Autodesk Inventor part; units mm, degrees
(part 2 of 2)
sketch "Sketch8" plane through (0, 0, 0) normal (0, 0, -1) x (-1, 0, 0)
  circle A0 centre (-9.53986, -23.285481) radius 1.25
  arc A1 (-7.169291, -24.867538) -> (-5.771961, -25.140998) centre (-5.772396, -21.436445) ccw
  arc A2 (-7.396071, -25.163424) -> (-7.169291, -24.867538) centre (-9.53986, -23.285481) ccw
  arc A3 (-6.768851, -26.441667) -> (-7.396071, -25.163424) centre (-10.346218, -27.404037) ccw
  arc A4 (-7.204522, -26.776355) -> (-6.768851, -26.441667) centre (-9.53986, -23.285481) ccw
  arc A5 (-8.277915, -25.840867) -> (-7.204522, -26.776355) centre (-5.352623, -23.567901) ccw
  arc A6 (-8.622256, -25.983722) -> (-8.277915, -25.840867) centre (-9.53986, -23.285481) ccw
  arc A7 (-8.718189, -27.404323) -> (-8.622256, -25.983722) centre (-12.297464, -26.449075) ccw
  arc A8 (-9.262835, -27.476335) -> (-8.718189, -27.404323) centre (-9.53986, -23.285481) ccw
  arc A9 (-9.724676, -26.129482) -> (-9.262835, -27.476335) centre (-6.054816, -25.623682) ccw
  arc A10 (-10.094312, -26.081028) -> (-9.724676, -26.129482) centre (-9.53986, -23.285481) ccw
  arc A11 (-10.887693, -27.263338) -> (-10.094312, -26.081028) centre (-13.509813, -24.646432) ccw
  arc A12 (-11.395376, -27.053379) -> (-10.887693, -27.263338) centre (-9.53986, -23.285481) ccw
  arc A13 (-11.121916, -25.65605) -> (-11.395376, -27.053379) centre (-7.690824, -27.052944) ccw
  arc A14 (-11.417803, -25.42927) -> (-11.121916, -25.65605) centre (-9.53986, -23.285481) ccw
  arc A15 (-12.696046, -26.05649) -> (-11.417803, -25.42927) centre (-13.658415, -22.479122) ccw
  arc A16 (-13.030733, -25.620818) -> (-12.696046, -26.05649) centre (-9.53986, -23.285481) ccw
  arc A17 (-12.095245, -24.547426) -> (-13.030733, -25.620818) centre (-9.822279, -27.472718) ccw
  arc A18 (-12.2381, -24.203085) -> (-12.095245, -24.547426) centre (-9.53986, -23.285481) ccw
  arc A19 (-13.658701, -24.107152) -> (-12.2381, -24.203085) centre (-12.703454, -20.527876) ccw
  arc A20 (-13.730714, -23.562506) -> (-13.658701, -24.107152) centre (-9.53986, -23.285481) ccw
  arc A21 (-12.383861, -23.100664) -> (-13.730714, -23.562506) centre (-11.878061, -26.770525) ccw
  arc A22 (-12.335406, -22.731029) -> (-12.383861, -23.100664) centre (-9.53986, -23.285481) ccw
  arc A23 (-13.517717, -21.937648) -> (-12.335406, -22.731029) centre (-10.90081, -19.315528) ccw
  arc A24 (-13.307758, -21.429964) -> (-13.517717, -21.937648) centre (-9.53986, -23.285481) ccw
  arc A25 (-11.910428, -21.703424) -> (-13.307758, -21.429964) centre (-13.307323, -25.134517) ccw
  arc A26 (-11.683648, -21.407538) -> (-11.910428, -21.703424) centre (-9.53986, -23.285481) ccw
  arc A27 (-12.310868, -20.129295) -> (-11.683648, -21.407538) centre (-8.733501, -19.166926) ccw
  arc A28 (-11.875197, -19.794607) -> (-12.310868, -20.129295) centre (-9.53986, -23.285481) ccw
  arc A29 (-10.801804, -20.730095) -> (-11.875197, -19.794607) centre (-13.727096, -23.003062) ccw
  arc A30 (-10.457463, -20.58724) -> (-10.801804, -20.730095) centre (-9.53986, -23.285481) ccw
  arc A31 (-10.36153, -19.166639) -> (-10.457463, -20.58724) centre (-6.782255, -20.121887) ccw
  arc A32 (-9.816884, -19.094627) -> (-10.36153, -19.166639) centre (-9.53986, -23.285481) ccw
  arc A33 (-9.355043, -20.44148) -> (-9.816884, -19.094627) centre (-13.024903, -20.94728) ccw
  arc A34 (-8.985407, -20.489934) -> (-9.355043, -20.44148) centre (-9.53986, -23.285481) ccw
  arc A35 (-8.192026, -19.307624) -> (-8.985407, -20.489934) centre (-5.569907, -21.92453) ccw
  arc A36 (-7.684343, -19.517583) -> (-8.192026, -19.307624) centre (-9.53986, -23.285481) ccw
  arc A37 (-7.957803, -20.914912) -> (-7.684343, -19.517583) centre (-11.388896, -19.518018) ccw
  arc A38 (-7.661916, -21.141693) -> (-7.957803, -20.914912) centre (-9.53986, -23.285481) ccw
  arc A39 (-6.383673, -20.514472) -> (-7.661916, -21.141693) centre (-5.421304, -24.09184) ccw
  arc A40 (-6.048986, -20.950144) -> (-6.383673, -20.514472) centre (-9.53986, -23.285481) ccw
  arc A41 (-6.984474, -22.023537) -> (-6.048986, -20.950144) centre (-9.25744, -19.098244) ccw
  arc A42 (-6.841619, -22.367877) -> (-6.984474, -22.023537) centre (-9.53986, -23.285481) ccw
  arc A43 (-5.421018, -22.46381) -> (-6.841619, -22.367877) centre (-6.376265, -26.043086) ccw
  arc A44 (-5.349006, -23.008457) -> (-5.421018, -22.46381) centre (-9.53986, -23.285481) ccw
  arc A45 (-6.695858, -23.470298) -> (-5.349006, -23.008457) centre (-7.201659, -19.800437) ccw
  arc A46 (-6.744313, -23.839933) -> (-6.695858, -23.470298) centre (-9.53986, -23.285481) ccw
  arc A47 (-5.562003, -24.633314) -> (-6.744313, -23.839933) centre (-8.178909, -27.255434) ccw
  arc A48 (-5.771961, -25.140998) -> (-5.562003, -24.633314) centre (-9.53986, -23.285481) ccw
  circle A49 centre (-9.53986, -23.285481) radius 4.2
  circle A50 centre (-9.53986, -23.285481) radius 4.6
  point P0 (0, 0)
  dimension "d138" = 0.4
  constraints: 1 centre point, 1 coincident, 3 other
extrude "Extrusion10" add sketch "Sketch8" against normal blind 1.6 contours A2 A3 A4 A5 A6 A7 A8 A9 A10 A11 A12 A13 A14 A15 A16 A17 A18 A19 A20 A21 A22 A23 A24 A25 A26 A27 A28 A29 A30 A31 A32 A33 A34 A35 A36 A37 A38 A39 A40 A41 A42 A43 A44 A45 A46 A47 A48 A1 | A1 A49 A3 A2 | A47 A46 A45 A49 | A49 A7 A6 A5 | A43 A42 A41 A49 | A49 A11 A10 A9 | A39 A38 A37 A49 | A49 A15 A14 A13 | A35 A34 A33 A49 | A49 A19 A18 A17 | A31 A30 A29 A49 | A49 A23 A22 A21 | A27 A26 A25 A49 | A50
fillet "Fillet1" radius 1 1 edges at (6.9456, -62.4312, 2)
sketch "Sketch10" plane through (0, 0, 9.3) normal (0, 0, 1) x (1, 0, 0)
  arc A0 (2, -23.367949) -> (-1, -25.1) centre (1, -25.1) ccw
  line L0 (-1, -33.180447) -> (-1, -25.1)
  spline S0 degree 2 poles (-1, -33.180447) (0.437273, -35.168536) (-1, -37.156626) knots 0 0 0 1 1 1 weights 1 1.44736842 1 construction
  line L1 (-1, -45.237072) -> (-1, -37.156626)
  line L2 (23.2, -66.431155) -> (0, -66.431155)
  line L3 (23.2, -6.5) -> (23.2, -66.431155)
  line L4 (27.5, -6.5) -> (23.2, -6.5)
  line L5 (27.5, 0) -> (27.5, -6.5)
  line L6 (0, 0) -> (27.5, 0)
  line L7 (0, -1) -> (0, 0)
  line L8 (2.5, -1) -> (0, -1)
  line L9 (2.5, -17.5) -> (2.5, -1)
  line L10 (0, -17.5) -> (2.5, -17.5)
  line L11 (0, -66.431155) -> (0, -17.5)
  arc A1 (4.201679, -29.771145) -> (17.167076, -26.804795) centre (12.35, -35.568116) ccw
  arc A2 (9.822706, -14.890244) -> (4.201679, -29.771145) centre (9.53986, -23.285481) ccw
  arc A3 (16.877474, -19.196543) -> (9.822706, -14.890244) centre (14.75, -14.75) ccw
  arc A4 (17.167076, -26.804795) -> (17.92577, -23.771799) centre (9.53986, -23.285481) ccw
  circle A5 centre (1.4, -30.121685) radius 0.6
  circle A6 centre (1.4, -41.467078) radius 0.6
  circle A7 centre (1.4, -30.121685) radius 2.229722
  circle A8 centre (1.4, -41.467078) radius 2.437856
  circle A9 centre (4, -46.805442) radius 3.5
  arc A10 (4.201679, -29.771145) -> (17.167076, -26.804795) centre (12.35, -35.568116) ccw
  arc A11 (9.822706, -14.890244) -> (4.201679, -29.771145) centre (9.53986, -23.285481) ccw
  circle A12 centre (10.75, -7.821797) radius 2.25
  arc A13 (17.92577, -23.771799) -> (17.265371, -19.98753) centre (18.75, -21.678203) ccw
  arc A14 (-1, -45.237072) -> (2, -46.969123) centre (1, -45.237072) ccw
  spline S1 degree 3 poles (3, -25.1) (3, -24.918932) (2.974149, -24.721818) (2.859633, -24.337077) (2.770851, -24.149343) (2.583999, -23.871436) (2.486925, -23.753405) (2.26049, -23.539413) (2.130887, -23.443517) (2, -23.367949) knots 0 0 0 0 0.29735014 0.29735014 0.59470027 0.59470027 0.79735014 0.79735014 1 1 1 1
  spline S2 degree 3 poles (2, -46.969123) (2.144805, -46.88552) (2.285887, -46.778364) (2.528279, -46.538397) (2.629848, -46.405654) (2.897307, -45.967482) (3, -45.573174) (3, -45.237072) knots 0 0 0 0 0.2241219 0.2241219 0.4482438 0.4482438 1 1 1 1
  line L12 (3, -25.1) -> (3, -45.237072)
  circle A15 centre (4, -46.805442) radius 1.2295
  arc A16 (17.265371, -19.98753) -> (16.877474, -19.196543) centre (9.53986, -23.285481) ccw
  point P0 (0, 0)
  point P1 (19.495918, -28.276795)
  dimension "d145" = 1.2
  dimension "d146" = 1.2
  dimension "d147" = 4.45944
  dimension "d148" = 4.87571
  dimension "d149" = 7
  dimension "d226" = 0.8
  dimension "d227" = 1
  dimension "d228" = 0.8
  dimension "d229" = 1
  constraints: 5 centre point, 4 tangent, 3 coincident, 2 end point, 1 vertical
  measures "d145" diameter of A5
  measures "d146" diameter of A6
  measures "d147" diameter of A7
  measures "d148" diameter of A8
  measures "d149" diameter of A9
  measures "d226" distance edge to line of A5 L11
  measures "d227" distance edge to line of A5 L12
  measures "d228" distance edge to line of A6 L11
  measures "d229" distance edge to line of A6 L12
hole "Hole7" at (1.4, -30.121685, 9.3) at (1.4, -41.467078, 9.3) direction (0, 0, -1) diameter 1.4 end through all
sketch "Sketch11" plane through (2.5, -17.5, 0) normal (-1, 0, 0) x (0, 0, 1)
  circle A0 centre (6, 7) radius 1.25 projected
  point P0 (0, 17.5)
hole "Hole8" at (2.5, -10.5, 6) direction (1, 0, 0) diameter 2.013 depth 8 thread size "M2.5x0.45" class "6H" standard "ISO Metric profile"
sketch "Sketch13" plane through (0, 0, 3.1) normal (0, 0, 1) x (1, 0, 0)
  arc A0 (6.999126, -27.120148) -> (13.495221, -25.633909) centre (12.35, -35.568116) ccw
  arc A1 (6.999126, -27.120148) -> (13.495221, -25.633909) centre (9.53986, -23.285481) ccw
  circle A2 centre (12.35, -35.568116) radius 5
  circle A3 centre (14.75, -14.75) radius 14.25
  circle A4 centre (14.7, -55.637072) radius 14
  circle A5 centre (18.375888, -31.102842) radius 2.5
  circle A6 centre (18.66148, -39.619685) radius 2.5
  circle A7 centre (6.235304, -31.225249) radius 2.5
  circle A8 centre (7.145272, -40.968191) radius 2.5
  point P0 (0, 0)
  dimension "d174" = 5
  dimension "d175" = 5
  dimension "d176" = 5
  dimension "d177" = 5
  dimension "d178" = 1.5
  constraints: 7 tangent, 4 centre point
  measures "d174" diameter of A5
  measures "d175" diameter of A6
  measures "d176" diameter of A8
  measures "d177" diameter of A7
hole "Hole10" at (18.375888, -31.102842, 3.1) at (18.66148, -39.619685, 3.1) at (7.145272, -40.968191, 3.1) at (6.235304, -31.225249, 3.1) direction (0, 0, -1) diameter 2.9 end through all counterbore diameter 5 counterbore depth 1.1 clearance for "Countersunk Flat Head Screw ISO 2009/7046" size "M2.5" standard "ISO"
sketch "Sketch14" plane through (0, 0, 3.1) normal (0, 0, 1) x (1, 0, 0)
  arc A0 (8.273536, -32.672871) -> (4.197072, -29.777627) centre (6.235304, -31.225249) ccw
  arc A1 (16.367259, -32.591266) -> (8.273536, -32.672871) centre (12.35, -35.568116) ccw
  arc A2 (20.384518, -29.614417) -> (16.367259, -32.591266) centre (18.375888, -31.102842) ccw
  arc A3 (20.384518, -29.614417) -> (13.495221, -25.633909) centre (12.35, -35.568116) ccw
  arc A4 (6.999126, -27.120148) -> (13.495221, -25.633909) centre (9.53986, -23.285481) ccw
  arc A5 (6.999126, -27.120148) -> (4.197072, -29.777627) centre (12.35, -35.568116) ccw
  arc A6 (20.765307, -40.970209) -> (16.557653, -38.269162) centre (18.66148, -39.619685) ccw
  arc A7 (20.765307, -40.970209) -> (20.384518, -29.614417) centre (12.35, -35.568116) ccw
  arc A8 (16.367259, -32.591266) -> (20.384518, -29.614417) centre (18.375888, -31.102842) ccw
  arc A9 (16.557653, -38.269162) -> (16.367259, -32.591266) centre (12.35, -35.568116) ccw
  arc A10 (5.410363, -42.768215) -> (8.880182, -39.168166) centre (7.145272, -40.968191) ccw
  arc A11 (16.557653, -38.269162) -> (20.765307, -40.970209) centre (18.66148, -39.619685) ccw
  arc A12 (8.880182, -39.168166) -> (16.557653, -38.269162) centre (12.35, -35.568116) ccw
  arc A13 (4.197072, -29.777627) -> (8.273536, -32.672871) centre (6.235304, -31.225249) ccw
  arc A14 (4.197072, -29.777627) -> (5.410363, -42.768215) centre (12.35, -35.568116) ccw
  arc A15 (8.880182, -39.168166) -> (5.410363, -42.768215) centre (7.145272, -40.968191) ccw
  arc A16 (8.273536, -32.672871) -> (8.880182, -39.168166) centre (12.35, -35.568116) ccw
  line L0 (16.303045, -29.705229) -> (15.145225, -31.422429)
  line L1 (19.109645, -33.492737) -> (17.129791, -34.100602)
  line L2 (15.416665, -39.517238) -> (16.686919, -41.153018)
  circle A17 centre (12.35, -35.568116) radius 5
  line L3 (10.27864, -40.118881) -> (9.420655, -42.00387)
  line L4 (7.878607, -37.805669) -> (6.026496, -38.732494)
  line L5 (9.471754, -31.479632) -> (8.279546, -29.786126)
  line L6 (5.549883, -33.629453) -> (7.541591, -34.197274)
  line L7 (17.217363, -36.712136) -> (19.23349, -37.186004)
  arc A18 (4.197072, -29.777627) -> (8.273536, -32.672871) centre (6.235304, -31.225249) ccw
  arc A19 (8.273536, -32.672871) -> (4.197072, -29.777627) centre (6.235304, -31.225249) ccw
  arc A20 (8.880182, -39.168166) -> (5.410363, -42.768215) centre (7.145272, -40.968191) ccw
  arc A21 (5.410363, -42.768215) -> (8.880182, -39.168166) centre (7.145272, -40.968191) ccw
  arc A22 (8.880182, -39.168166) -> (16.557653, -38.269162) centre (12.35, -35.568116) ccw
  arc A23 (16.557653, -38.269162) -> (20.765307, -40.970209) centre (18.66148, -39.619685) ccw
  arc A24 (16.367259, -32.591266) -> (20.384518, -29.614417) centre (18.375888, -31.102842) ccw
  arc A25 (16.367259, -32.591266) -> (8.273536, -32.672871) centre (12.35, -35.568116) ccw
  arc A26 (5.410363, -42.768215) -> (20.765307, -40.970209) centre (12.35, -35.568116) ccw
  point P0 (0, 0)
  point P1 (16.367259, -32.591266)
  point P2 (16.367259, -32.591266)
  point P3 (17.217363, -36.712136)
  point P4 (16.557653, -38.269162)
  point P5 (16.557653, -38.269162)
  point P6 (16.557653, -38.269162)
  point P7 (8.880182, -39.168166)
  point P8 (8.880182, -39.168166)
  point P9 (7.878607, -37.805669)
  point P10 (6.026496, -38.732494)
  point P11 (7.541591, -34.197274)
  point P12 (8.273536, -32.672871)
  point P13 (8.273536, -32.672871)
  point P14 (9.471754, -31.479632)
  constraints: 18 point on circle, 16 end point, 8 tangent, 2 line through centre, 12 other
extrude "Extrusion12" cut sketch "Sketch14" against normal up to surface (1.1 mm away) contours A0 L5 A1 | A16 L6 A13 | L0 A2 A1 | A16 A15 L4 | A8 L1 A9 | A6 A9 L7
sketch "Sketch15" plane through (0, 0, 0) normal (0, 1, 0) x (1, 0, 0)
  line L0 (27.5, 0) -> (0, 0) projected
  line L1 (0, 0) -> (0, -9.3) projected
  line L2 (0, -9.3) -> (27.5, -9.3) projected
  line L3 (27.5, 0) -> (27.5, -9.3) projected
  line L4 (27.5, 0) -> (0, 0) projected
  line L5 (23.2, 0) -> (23.2, -9.3)
  line L6 (3, -9.3) -> (3, 0)
  line L7 (0, 0) -> (0, -9.3) projected
  circle A0 centre (18.15, -3.25) radius 3.25
  circle A1 centre (8.05, -3.25) radius 3.25
  line L8 (13.1, 0) -> (13.1, -9.3)
  dimension "d195" = 4.3
  dimension "d196" = 3
  dimension "d197" = 6.5
  dimension "d198" = 6.5
  dimension "d202" = 5.05
  dimension "d203" = 5.05
  dimension "d206" = 10.1
  dimension "d207" = 10.1
  dimension "d208" = 5.05
  dimension "d209" = 5.05
  constraints: 6 end point, 6 point on line, 2 centre point, 2 perpendicular, 2 tangent, 1 parallel
  measures "d195" distance between parallel lines of L3 L5
  measures "d196" distance between parallel lines of L1 L6
  measures "d197" diameter of A0
  measures "d198" diameter of A1
  measures "d202" distance from line of A0.centre L5
  measures "d203" distance from line of L6 A1.centre
  measures "d206" distance between parallel lines of L6 L8
  measures "d207" distance between parallel lines of L5 L8
  measures "d208" distance from line of L8 A0.centre
  measures "d209" distance from line of A1.centre L8
hole "Hole11" at (18.15, 0, 3.25) at (8.05, 0, 3.25) direction (0, -1, 0) diameter 2.459 depth 6.5 thread size "M3x0.5" class "6H" standard "ISO Metric profile"
ref_plane "Work Plane4" through (0, 1, 0) normal (0, 1, 0) x (1, 0, 0)
sketch "Sketch16" plane through (0, 1, 0) normal (0, 1, 0) x (1, 0, 0)
  circle A0 centre (18.15, -3.25) radius 1.2295 projected
  circle A1 centre (8.05, -3.25) radius 1.2295 projected
  point P0 (0, 0)
hole "Hole12" at (8.05, 1, 3.25) at (18.15, 1, 3.25) direction (0, -1, 0) diameter 0.1 depth 5 countersink diameter 7 countersink angle 90
fillet "Fillet2" radius 1 6 edges at (17.2174, -36.7121, 2.55) (7.8786, -37.8057, 2.55) (7.5416, -34.1973, 2.55) (15.1452, -31.4224, 2.55) (17.1298, -34.1006, 2.55) (9.4718, -31.4796, 2.55)
fillet "Fillet3" radius 3 3 edges at (6.7245, -65.4312, 2) (23.2, -46.6814, 2) (23.2, -50.8312, 2)
body "Solid2"
